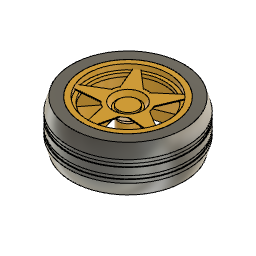
roue (Autodesk Fusion 360 design; units mm, degrees)
Autodesk Fusion 360 part; units mm, degrees
note: some values were not read from the file. Chosen so that the rebuilt part matches the saved one: which bodies a step acts on; which face or edge a step refers to. Set by a fixed rule: which sketch regions a step uses.
sketch "Esquisse1" plane through (0, 0, 0) normal (1, 0, 0) x (0, 1, 0)
  circle A0 centre (0, 0) radius 34.5
  line L0 (-34.5, 2.9995) -> (-34.5, 4)
  line L1 (-34.5, 4) -> (-34.5, 2)
  line L2 (-34.5, 2) -> (-33.5, 2)
  line L3 (-33.5, 2) -> (-33.5, 4)
  line L4 (-33.5, 4) -> (-34.5, 4)
  line L5 (-33.5, -2) -> (-33.5, -4)
  line L6 (-34.5, -2) -> (-33.5, -2)
  line L7 (-33.5, -4) -> (-34.5, -4)
  line L8 (0, 0) -> (0, 13)
  line L9 (0, 13) -> (0, 0)
  line L10 (0, 0) -> (0, -13)
  line L11 (0, -13) -> (-34, -13)
  line L12 (-34, -13) -> (-34, 13)
  line L13 (-34, 13) -> (0, 13)
  line L14 (-34, 13) -> (-26, 13)
  line L15 (-26, -13) -> (-26, 13)
  dimension "d1" = 69
  dimension "d11" = 1
  constraint coincident A0.centre L8.start
  constraint perpendicular L0 L4
  constraint vertical L8
  constraint parallel L8 L9
  constraint parallel L9 L10
  constraint perpendicular L10 L11
  constraint perpendicular L11 L12
  constraint perpendicular L8 L13
  constraint coincident L13 L14.end
  constraint perpendicular L14 L15
  measures "d1" diameter of A0
  measures "d11" distance of L1.end L2.end
revolve "Révolution3" add sketch "Esquisse1" angle 360 about axis through (0, 0, -11.9026) along (0, 0, 1) contours A0 L2 L3 L4 L5 L6 L7 L11 L12 L13 L14 L15 makes body 1
sketch "Esquisse3" plane through (0, 0, 0) normal (0, 0, 1) x (1, 0, 0)
cylinder "CylinderPrimitive2" add diameter 51.884 height 13 placed x (1, 0, 0) y (0, 1, 0) z (0, 0, 1) at (0, 0, 0) separate body makes body 2
extrude "Extrusion3" add 1 faces at (-5.2205, 3.9446, 0) along direction (0, 0, -1) blind 13 on bodies 2 bodies 2
hole "Perçage2" at (0, 0, 14.1) direction (0, 0, -1) diameter 46 depth 39.815 tip angle 118 bodies 2
ref_plane "Plan de construction1" through (0, 0, 8) normal (0, 0, 1) x (1, 0, 0)
sketch "Esquisse5" plane through (0, 0, 8) normal (0, 0, 1) x (1, 0, 0)
cylinder "CylinderPrimitive3" add diameter 46 height 2 placed x (1, 0, 0) y (0, 1, 0) z (0, 0, 1) at (0, 0, 8) bodies 2
hole "Perçage3" at (0, 0, 10) direction (0, 0, -1) diameter 42 depth 39.815 tip angle 118 bodies 2
ref_plane "Plan de construction3" through (0, 0, -18) normal (0, 0, 1) x (1, 0, 0)
cylinder "CylinderPrimitive4" add diameter 11 height 27 placed x (1, 0, 0) y (0, 1, 0) z (0, 0, 1) at (0, 0, -18) separate body makes body 3
hole "Perçage4" at (0, 0, -18) direction (0, 0, 1) diameter 6 depth 1.05 tip angle 180 bodies 3
sketch "Esquisse7" plane through (0, 0, -16.95) normal (0, 0, -1) x (1, 0, 0)
  circle A0 centre (0, 0) radius 3
  line L0 (1.7, 0) -> (1.7, -2.4718)
  line L1 (1.7, 0) -> (1.7, 2.4718)
  line L2 (-1.7, -2.4718) -> (-1.7, 2.4718)
  constraint coincident A0 L0.end
  constraint coincident A0 L1.end
  constraint coincident A0 L2.start
  constraint coincident A0 L2.end
extrude "Extrusion4" cut sketch "Esquisse7" against normal blind 9.95 contours A0 L0 L1 L2 bodies 3
ref_plane "Plan de construction4" through (0, 0, 3.5) normal (0, 0, 1) x (1, 0, 0)
split "Scinder1" by plane through (0, 0, 3.5) normal (0, 0, 1) bodies 3 makes body 4 at (5.4727, -0.5476, 7.1667)
extrude "Extrusion5" add 1 faces at (0.6698, -1.7066, 3.5) along direction (0, 0, 1) blind 7 draft 38.157 on bodies 4 bodies 4 3
ref_plane "Plan de construction5" through (0, 0, 6.5) normal (0, 0, 1) x (1, 0, 0)
sketch "Esquisse9" plane through (0, 0, 6.5) normal (0, 0, 1) x (1, 0, 0)
  circle A0 centre (0, 0) radius 5.5
  dimension "d53" = 11
  constraint coincident A0.centre origin
  measures "d53" diameter of A0
extrude "Extrusion6" cut sketch "Esquisse9" along normal blind 7 draft 38.157 bodies 4
ref_plane "Plan de construction6" through (0, 0, 6) normal (0, 0, 1) x (1, 0, 0)
cylinder "CylinderPrimitive5" add diameter 15 height 2 placed x (1, 0, 0) y (0, 1, 0) z (0, 0, 1) at (0, 0, 6) bodies 4
cylinder "CylinderPrimitive6" add diameter 11 height 1 placed x (1, 0, 0) y (0, 1, 0) z (0, 0, 1) at (0, 0, 8) bodies 4
sketch "Esquisse13" plane through (0, 0, 10.5) normal (0, 0, 1) x (-1, 0, 0)
  circle A0 centre (0, 0) radius 8.6428
  circle A1 centre (0, 0) radius 11
  line L0 (5, 8.66) -> (-5, 8.66)
  line L1 (0, 30) -> (5, 8.66)
  line L2 (0, 30) -> (-5, 8.66)
  line L3 (0, 30) -> (5, 8.66)
  dimension "d61" = 8.66
  constraint horizontal L0
  constraint parallel L1 L3
  measures "d61" distance of A0.centre L0
extrude "Extrusion7" add sketch "Esquisse13" against normal blind 0.5 separate body contours A1 L0 L1 L2 L3 | A1 L1 L2 L3 picked at (0, 9.44) makes body 5
pattern_circular "Réseau C1" count 5 over 360 about axis through (0, 0, 1.75) along (0, 0, 1) of bodies 5 makes body 6 at (15.8166, -5.1391, 10.5) makes body 7 at (9.7752, 13.4544, 10.5) makes body 8 at (-9.7752, 13.4544, 10.5) makes body 9 at (-15.8166, -5.1391, 10.5)
combine "Combiner1" operation add target body 5 tool bodies 6 7 8 9 4
sketch "Esquisse14" plane through (0, 0, 0) normal (1, 0, 0) x (0, 1, 0)
  line L0 (0, 10) -> (-25, 10)
  line L1 (-25, 10) -> (-25, 0)
  line L2 (-25, 0) -> (0, 10)
  constraint horizontal L0
  constraint perpendicular L0 L1
extrude "Extrusion8" add sketch "Esquisse14" along normal blind 0.25 and the other way blind 0.25 separate body makes body 10
split "Scinder2" by face at (8.5699, 1.2917, 7.5303) of body 5 bodies 10 makes body 11 at (-0.25, -20.2014, 6.6667)
delete_body "RemoveBody1" bodies 10
pattern_circular "Réseau C2" count 5 over 360 about axis through (0, 0, -18) along (0, 0, 1) of bodies 11 makes body 12 at (19.1354, -6.4803, 6.6667) makes body 13 at (12.0763, 16.1963, 6.6667) makes body 14 at (-11.6718, 16.4902, 6.6667) makes body 15 at (-19.2899, -6.0048, 6.6667)
combine "Combiner2" operation add target body 5 tool bodies 14 15 13 12 11
named bodies: "Pneu", "Support pneu", "Arbre", "Arbre (1)", "Arbre et moyeu"
